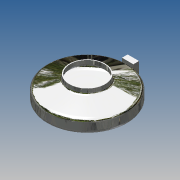
# Autodesk Inventor part: inlineFan
Saved by Autodesk Inventor 2014 SP1 (Build 180222100, 222)
## iProperties
Created: 2014-08-21
Part Number: inlineFan
Material: Nickel-Copper Alloy 400
Document SubType Name: Modeling
Designer: Dave
Density: 8.83 g/cm^3
Appearance: Chrome - Polished
Mass: 8598.39 g
Surface Area: 4893.66 cm^2
Volume: 973.77 cm^3
Author: Dave
Autodesk Inventor part; units mm, degrees
ref_plane "YZ Plane" through (0, 0, 0) normal (1, 0, 0) x (0, 1, 0)
ref_plane "XZ Plane" through (0, 0, 0) normal (0, 1, 0) x (-1, 0, 0)
ref_plane "XY Plane" through (0, 0, 0) normal (0, 0, 1) x (1, 0, 0)
sketch "Sketch1" plane through (0, 0, 0) normal (1, 0, 0) x (0, 1, 0)
  line L0 (0, 0) -> (13.7626, 0)
  line L1 (26.4143, 11.5931) -> (33.2408, 89.6203)
  line L2 (45.8924, 101.2134) -> (75.31, 101.2134)
  arc A0 (45.8924, 101.2134) -> (33.2408, 89.6203) centre (45.8924, 88.5134) ccw
  arc A1 (87.5916, 91.7463) -> (75.31, 101.2134) centre (75.31, 88.5134) ccw
  arc A2 (13.7626, 0) -> (26.4143, 11.5931) centre (13.7626, 12.7) ccw
  line L3 (87.5916, 91.7463) -> (109.2504, 9.4671)
  line L4 (121.532, 0) -> (137.1424, 0)
  arc A3 (109.2504, 9.4671) -> (121.532, 0) centre (121.532, 12.7) ccw
  line L5 (137.1424, 3.81) -> (121.532, 3.81)
  arc A4 (112.9349, 10.437) -> (121.532, 3.81) centre (121.532, 12.7) ccw
  line L6 (112.9349, 10.437) -> (91.2761, 92.7162)
  arc A5 (91.2761, 92.7162) -> (75.31, 105.0234) centre (75.31, 88.5134) ccw
  line L7 (75.31, 105.0234) -> (45.8924, 105.0234)
  arc A6 (45.8924, 105.0234) -> (29.4453, 89.9523) centre (45.8924, 88.5134) ccw
  line L8 (29.4453, 89.9523) -> (22.6188, 11.9252)
  arc A7 (13.7626, 3.81) -> (22.6188, 11.9252) centre (13.7626, 12.7) ccw
  line L9 (13.7626, 3.81) -> (0, 3.81)
  line L10 (137.1424, 3.81) -> (137.1424, 0)
  line L11 (0, 3.81) -> (0, 0)
  line L12 (9.8653, -76.2) -> (185.5635, -76.2) construction
  point P0 (25.4, 0)
  point P1 (34.255, 101.2134)
  point P2 (85.055, 101.2134)
  point P3 (111.7424, 0)
  dimension "d0" = 25.4
  dimension "d1" = 101.6
  dimension "d2" = 95
  dimension "d3" = 50.8
  dimension "d4" = 95
  dimension "d7" = 12.7
  dimension "d9" = 25.4
  dimension "d10" = 12.7
  dimension "d11" = 3.81
  dimension "d12" = 76.2
  constraints: 26 end point, 16 point on circle, 8 centre point, 8 tangent, 7 point on line, 5 parallel, 2 perpendicular, 1 equal radius, 1 horizontal, 8 other
  measures "d0" distance of L0.start point (25.4, 0)
  measures "d1" distance of point (25.4, 0) point (34.255, 101.213)
  measures "d2" angle of L1 L0
  measures "d3" distance of point (34.255, 101.213) point (85.055, 101.213)
  measures "d4" angle of L1 L2
  measures "d7" radius of A0
  measures "d9" distance of point (111.742, 0) L4.end
  measures "d10" radius of A3
  measures "d11" distance between parallel lines of L3 L6
  measures "d12" distance between parallel lines of L12 L0
revolve "Revolution1" add sketch "Sketch1" angle 360 about axis through (0, 9.8653, -76.2) along (0, 1, 0)
sketch "Sketch3" plane through (0, 0, 0) normal (1, 0, 0) x (0, 1, 0)
  line L0 (45.8782, -257.0249) -> (96.6782, -257.0249)
  line L1 (96.6782, -257.0249) -> (96.6782, -282.4249)
  line L2 (96.6782, -282.4249) -> (45.8782, -282.4249)
  line L3 (45.8782, -282.4249) -> (45.8782, -257.0249)
  point P0 (0, 0)
  dimension "d14" = 50.8
  dimension "d15" = 25.4
  constraints: 8 end point, 2 parallel, 1 horizontal, 1 perpendicular
  measures "d14" distance of L1.end L2.end
  measures "d15" distance of L0.end L1.end
extrude "Extrusion1" add sketch "Sketch3" along normal mid plane 50.8
body "Solid1"
